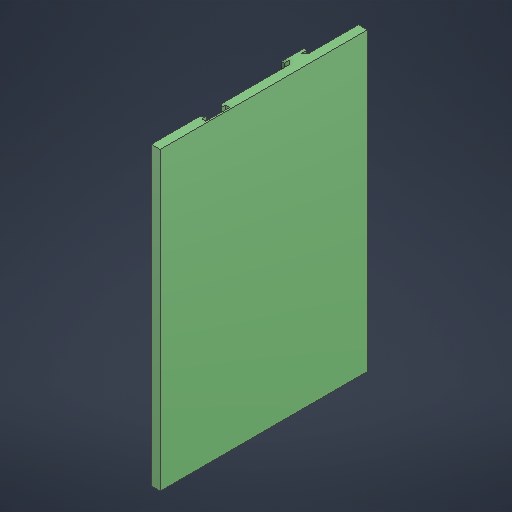
# Autodesk Inventor part: Edge
Saved by Autodesk Inventor 2027 (Build 310192060, 192F)
## iProperties
Created: 2026-06-12
Part Number: Edge
Material: Ogólny
Document SubType Name: Modeling
Designer: User
Density: 1 g/cm^3
Appearance: Domyślna
Author: User
Autodesk Inventor part; units mm, degrees
ref_plane "YZ Plane" through (0, 0, 0) normal (1, 0, 0) x (0, 1, 0)
ref_plane "XZ Plane" through (0, 0, 0) normal (0, 1, 0) x (-1, 0, 0)
ref_plane "XY Plane" through (0, 0, 0) normal (0, 0, 1) x (1, 0, 0)
sketch "Szkic1" plane through (0, 0, 0) normal (0, 1, 0) x (-1, 0, 0)
  line L0 (0, 3.5607) -> (1.0607, 2.5) construction
  line L1 (1.0607, 2.5) -> (1.0607, 4) construction
  line L2 (1.0607, 4) -> (2.4607, 4) construction
  line L3 (2.4607, 4) -> (2.4607, 0) construction
  line L4 (2.4607, 0) -> (0, 0) construction
  line L5 (0, -3.5607) -> (1.0607, -2.5) construction
  line L6 (2.4607, -4) -> (2.4607, 0) construction
  line L7 (1.0607, -4) -> (2.4607, -4) construction
  line L8 (1.0607, -2.5) -> (1.0607, -4) construction
  line L9 (0, 3.5607) -> (0, -3.5607)
  line L10 (0, 3.5607) -> (-1.0607, 2.5)
  line L11 (-1.0607, 2.5) -> (-1.0607, 4)
  line L12 (-1.0607, 4) -> (-2.4607, 4)
  line L13 (-2.4607, 4) -> (-2.4607, 0)
  line L14 (-2.4607, 0) -> (0, 0) construction
  line L15 (-2.4607, -4) -> (-2.4607, 0)
  line L16 (-1.0607, -4) -> (-2.4607, -4)
  line L17 (0, -3.5607) -> (-1.0607, -2.5)
  line L18 (-1.0607, -2.5) -> (-1.0607, -4)
  line L19 (0, 3.5607) -> (0, 23.5607)
  line L20 (0, 3.5607) -> (20, 3.5607) construction
  line L21 (0, 23.5607) -> (0, -46.4393)
  line L22 (0, 23.5607) -> (70, 23.5607) construction
  line L23 (0, -26.4393) -> (-1.0607, -27.5) construction
  line L24 (-1.0607, -27.5) -> (-1.0607, -26) construction
  line L25 (0, -33.5607) -> (-1.0607, -32.5) construction
  line L26 (-1.0607, -32.5) -> (-1.0607, -34) construction
  line L27 (-1.0607, -26) -> (-2.4607, -26) construction
  line L28 (-2.4607, -26) -> (-2.4607, -30) construction
  line L29 (-2.4607, -34) -> (-2.4607, -30) construction
  line L30 (-1.0607, -34) -> (-2.4607, -34) construction
  line L31 (-2.4607, -30) -> (0, -30) construction
  line L32 (2.4607, -30) -> (0, -30) construction
  line L33 (0, -26.4393) -> (1.0607, -27.5)
  line L34 (1.0607, -27.5) -> (1.0607, -26)
  line L35 (1.0607, -26) -> (2.4607, -26)
  line L36 (2.4607, -26) -> (2.4607, -30)
  line L37 (0, -26.4393) -> (20, -26.4393) construction
  line L38 (0, -33.5607) -> (1.0607, -32.5)
  line L39 (2.4607, -34) -> (2.4607, -30)
  line L40 (1.0607, -34) -> (2.4607, -34)
  line L41 (1.0607, -32.5) -> (1.0607, -34)
  line L42 (0, 23.5607) -> (-3, 23.5607)
  line L43 (-3, 23.5607) -> (-3, -46.4393)
  line L44 (-3, -46.4393) -> (0, -46.4393)
  line L45 (0, -46.4393) -> (0, 23.5607)
  point P0 (0, 0)
  point P1 (1.2303, 0)
  point P2 (-1.2303, 0)
  point P3 (-1.2303, -30)
  point P4 (1.2303, -30)
  point P5 (0, -3.5607)
  dimension "d0" = 1.5
  dimension "d1" = 1.5
  dimension "d2" = 1.4
  dimension "d3" = 4
  dimension "d4" = 45
  dimension "d5" = 20
  dimension "d6" = 90
  dimension "d7" = 70
  dimension "d8" = 90
  dimension "d11" = 30
  dimension "d16" = 3
  constraints: 92 end point, 11 symmetric about line, 3 horizontal, 3 perpendicular, 3 vertical, 2 parallel, 1 collinear, 1 midpoint, 39 other
  measures "d0" distance of L0.start L0.end
  measures "d1" distance of L0.end L1.end
  measures "d2" distance of L1.end L2.end
  measures "d3" distance of L2.end L3.end
  measures "d4" angle of L8 L5
  measures "d5" distance of L0.start L19.end
  measures "d6" angle of L20 L19
  measures "d7" distance of L19.end L21.end
  measures "d8" angle of L21 L22
  measures "d11" distance of L10.end L23.end
  measures "d16" distance of L44.end L43.end
extrude "Wyciągnięcie proste1" add sketch "Szkic1" along normal blind 100 contours L10 L11 L12 L13 L15 L16 L18 L17 L21 L44 L43 L42 L19 | L33 L34 L35 L36 L39 L40 L41 L38 L21
offset faces "Rozmiar1" outward -0.2 faces at (-2.4607, 33.3333, -31.3333) (-1.994, 33.3333, -26) (-1.5273, 33.3333, -34) (-0.3536, 33.3333, -33.2071) (-0.7071, 33.3333, -27.1464) (-1.0607, 33.3333, -26.5) (-1.0607, 33.3333, -33)
move faces "Przesuń2" translate (0, 0, -3.56) faces at (1, 33.3333, 23.5607) (2, 33.3333, -46.4393)
